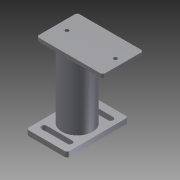
# Autodesk Inventor part: Lickport_Stand
Saved by Autodesk Inventor 2012 SP2 (Build 160219200, 219)
## iProperties
Created: 2014-11-07
Part Number: Lickport_Stand
Material: Default
Document SubType Name: Modeling
Designer: zhaox11
Density: 1 g/cm^3
Author: zhaox11
Autodesk Inventor part; units mm, degrees
ref_plane "YZ Plane" through (0, 0, 0) normal (1, 0, 0) x (0, 1, 0)
ref_plane "XZ Plane" through (0, 0, 0) normal (0, 1, 0) x (-1, 0, 0)
ref_plane "XY Plane" through (0, 0, 0) normal (0, 0, 1) x (1, 0, 0)
sketch "Sketch2" plane through (0, 0, 0) normal (0, 1, 0) x (-1, 0, 0)
  line L0 (-25.4, 38.1) -> (25.4, 38.1)
  line L1 (25.4, 38.1) -> (25.4, -38.1)
  line L2 (25.4, -38.1) -> (-25.4, -38.1)
  line L3 (-25.4, -38.1) -> (-25.4, 38.1)
  point P0 (0, 0)
  dimension "d0" = 50.8
  dimension "d1" = 76.2
  dimension "d2" = 25.4
  dimension "d3" = 38.1
  constraints: 8 end point, 2 parallel, 1 horizontal, 1 perpendicular
  measures "d0" distance of L1.end L2.end
  measures "d1" distance of L0.end L1.end
  measures "d2" distance from line of point (0, 0) L1
  measures "d3" distance from line of point (0, 0) L2
extrude "Extrusion1" add sketch "Sketch2" against normal blind 6.35
sketch "Sketch3" plane through (0, 0, 0) normal (0, 1, 0) x (1, 0, 0)
  circle A0 centre (0, 0) radius 19.05
  dimension "d6" = 38.1
  constraints: 1 centre point, 1 coincident
  measures "d6" diameter of A0
extrude "Extrusion2" add sketch "Sketch3" along normal blind 88.9
sketch "Sketch4" plane through (0, 0, 0) normal (0, 1, 0) x (1, 0, 0)
  circle A0 centre (0, 0) radius 19.05 projected
  line L0 (-15.875, 28.829) -> (15.875, 28.829)
  line L1 (15.875, 28.829) -> (15.875, 21.971)
  line L2 (15.875, 21.971) -> (-15.875, 21.971)
  line L3 (-15.875, 21.971) -> (-15.875, 28.829)
  line L4 (-15.875, -21.971) -> (15.875, -21.971)
  line L5 (15.875, -21.971) -> (15.875, -28.829)
  line L6 (15.875, -28.829) -> (-15.875, -28.829)
  line L7 (-15.875, -28.829) -> (-15.875, -21.971)
  line L8 (-15.875, 25.4) -> (15.875, 25.4)
  line L9 (-15.875, -25.4) -> (15.875, -25.4)
  circle A1 centre (-15.875, 25.4) radius 3.429
  circle A2 centre (15.875, 25.4) radius 3.429
  circle A3 centre (15.875, -25.4) radius 3.429
  circle A4 centre (-15.875, -25.4) radius 3.429
  dimension "d10" = 6.858
  dimension "d11" = 6.858
  dimension "d12" = 25.4
  dimension "d14" = 25.4
  dimension "d15" = 31.75
  dimension "d16" = 31.75
  dimension "d17" = 15.875
  dimension "d18" = 15.875
  constraints: 20 end point, 4 coincident, 4 midpoint, 4 parallel, 4 vertical alignment, 2 horizontal, 2 perpendicular, 8 other
  measures "d10" distance of L0.end L1.end
  measures "d11" distance of L4.end L5.end
  measures "d12" distance from line of A0.centre L8
  measures "d14" distance from line of A0.centre L9
  measures "d15" distance of L0.start L0.end
  measures "d16" distance of L5.end L6.end
  measures "d17" distance from line of A0.centre L3
  measures "d18" distance from line of A0.centre L7
sketch "Sketch5" plane through (0, 88.9, 0) normal (0, 1, 0) x (1, 0, 0)
  circle A0 centre (0, 0) radius 19.05 projected
  line L0 (-25.4, 25.4) -> (57.15, 25.4)
  line L1 (57.15, 25.4) -> (57.15, -25.4)
  line L2 (57.15, -25.4) -> (-25.4, -25.4)
  line L3 (-25.4, -25.4) -> (-25.4, 25.4)
  dimension "d19" = 50.8
  dimension "d20" = 82.55
  dimension "d21" = 25.4
  dimension "d22" = 25.4
  constraints: 8 end point, 2 parallel, 1 horizontal, 1 perpendicular
  measures "d19" distance of L2.end L0.start
  measures "d20" distance of L0.start L0.end
  measures "d21" distance from line of A0.centre L3
  measures "d22" distance from line of A0.centre L0
extrude "Extrusion3" add sketch "Sketch5" along normal blind 4.445 contours A0 | L0 L1 L2 L3
sketch "Sketch6" plane through (0, 93.345, 0) normal (0, 1, 0) x (1, 0, 0)
  line L0 (-25.4, -25.4) -> (-25.4, 25.4) projected
  circle A0 centre (-12.7, 0) radius 2.159
  circle A1 centre (47.625, 0) radius 2.159
  point P0 (0, 0)
  dimension "d25" = 4.318
  dimension "d26" = 12.7
  dimension "d27" = 4.318
  dimension "d28" = 60.325
  constraints: 2 centre point
  measures "d25" diameter of A0
  measures "d26" distance from line of L0 A0.centre
  measures "d27" diameter of A1
  measures "d28" distance of A1.centre A0.centre
extrude "Extrusion4" cut sketch "Sketch6" against normal blind 10.16
extrude "Extrusion5" cut sketch "Sketch4" against normal blind 6.35 contours A1 L8 L3 | L0 A2 L8 A1 | L3 A1 | A2 L1 | L1 L8 A2 | L8 A1 L3 | L8 A2 L2 A1 | L1 A2 L8 | A4 L9 L7 | L4 A3 L9 A4 | L7 A4 | A3 L5 | L5 L9 A3 | L9 A4 L7 | L9 A3 L6 A4 | L5 A3 L9
fillet "Fillet1" radius 3.175 8 edges at (-25.4, -3.175, 38.1) (25.4, -3.175, 38.1) (25.4, -3.175, -38.1) (-25.4, -3.175, -38.1) (57.15, 91.1225, -25.4) (-25.4, 91.1225, -25.4) (57.15, 91.1225, 25.4) (-25.4, 91.1225, 25.4)
sketch "Sketch7" plane through (0, 93.345, 0) normal (0, 1, 0) x (1, 0, 0)
  arc A0 (-25.4, -22.225) -> (-22.225, -25.4) centre (-22.225, -22.225) ccw projected
  line L0 (53.975, -25.4) -> (-22.225, -25.4) projected
  arc A1 (53.975, -25.4) -> (57.15, -22.225) centre (53.975, -22.225) ccw projected
  line L1 (57.15, 22.225) -> (57.15, -22.225) projected
  arc A2 (57.15, 22.225) -> (53.975, 25.4) centre (53.975, 22.225) ccw projected
  line L2 (-22.225, 25.4) -> (53.975, 25.4) projected
  arc A3 (-22.225, 25.4) -> (-25.4, 22.225) centre (-22.225, 22.225) ccw projected
  line L3 (-25.4, -22.225) -> (-25.4, 22.225) projected
  circle A4 centre (47.625, 0) radius 2.159 projected
  circle A5 centre (-12.7, 0) radius 2.159 projected
  point P0 (0, 0)
  dimension "d34" = 60.325
  measures "d34" distance of A4.centre A5.centre
thread "Thread1" size "10-24 UNC" class "2B" standard "ANSI Unified Screw Threads" full length
equation "\"d3\" = 0.5 * d1"
equation "\"d16\" = d15"
equation "\"d17\" = 0.5 * d15"
equation "\"d18\" = d17"
equation "\"d22\" = 0.5 * d19"
body "Solid1"
